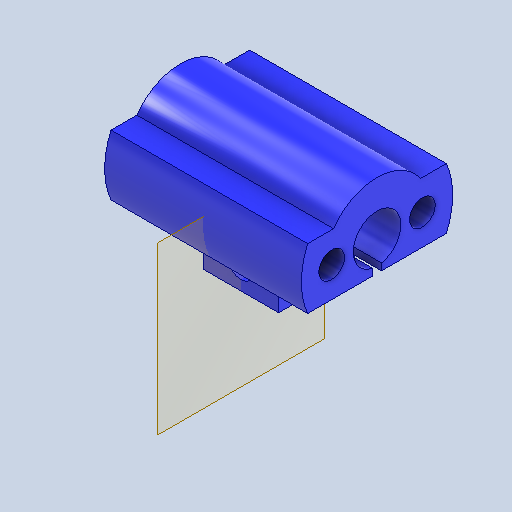
# Autodesk Inventor part: セットカラ―
Saved by Autodesk Inventor 2024 (Build 280153000, 153)
## iProperties
Created: 2020-01-17
Part Number: セットカラ―
Material: ABS プラスチック
Document SubType Name: Modeling
Designer: Hagihara Yuya
Density: 1.06 g/cm^3
Appearance: 青 - 壁塗料 - 光沢
Author: Hagihara Yuya
Autodesk Inventor part; units mm, degrees
ref_plane "YZ Plane" through (0, 0, 0) normal (1, 0, 0) x (0, 1, 0)
ref_plane "XZ Plane" through (0, 0, 0) normal (0, 1, 0) x (-1, 0, 0)
ref_plane "XY Plane" through (0, 0, 0) normal (0, 0, 1) x (1, 0, 0)
sketch "スケッチ1" plane through (0, 0, 0) normal (1, 0, 0) x (0, 1, 0)
  circle A0 centre (0, 0) radius 3.15
  circle A1 centre (0, 0) radius 7
  line L0 (0, 5) -> (-10, 5)
  line L1 (-10, 5) -> (-10, -5)
  line L2 (-10, -5) -> (0, -5)
  line L3 (0, -5) -> (0, 5) construction
  line L4 (-10, 0.6) -> (0, 0.6)
  line L5 (0, 0.6) -> (0, -0.6)
  line L6 (0, -0.6) -> (-10, -0.6)
  line L7 (-10, -0.6) -> (-10, 0.6)
  line L8 (4, 10) -> (-4, 10) construction
  line L9 (-4, 10) -> (-4, -10)
  line L10 (-4, -10) -> (4, -10) construction
  line L11 (4, -10) -> (4, 10)
  line L12 (4, 10) -> (-4, -10) construction
  line L13 (-4, 10) -> (4, -10) construction
  arc A2 (4, 9.1652) -> (-4, 9.1652) centre (0, 0) ccw
  arc A3 (-4, -9.1652) -> (4, -9.1652) centre (0, 0) ccw
  point P0 (-11, 3.3541)
  point P1 (-11, -3.3541)
  point P2 (-4.899, 5)
  point P3 (-4.899, -5)
  point P4 (-3.0923, 0.6)
  point P5 (-3.0923, -0.6)
  point P6 (-6.9742, -0.6)
  point P7 (-6.9742, 0.6)
  point P8 (0, -3.15)
  point P9 (0, 3.15)
  point P10 (0, 0.6)
  point P11 (-4, -5)
  point P12 (4, -5.7446)
  point P13 (4, 5.7446)
  point P14 (-4, 5)
  dimension "d0" = 6.3
  dimension "d1" = 14
  dimension "d2" = 5
  dimension "d3" = 5
  dimension "d4" = 10
  dimension "d18" = 1.2
  dimension "d19" = 0.6
  dimension "d45" = 8
  dimension "d46" = 20
  constraints: 28 end point, 6 parallel, 6 point on line, 4 centre point, 4 coincident, 4 point on circle, 3 horizontal, 3 midpoint, 3 perpendicular, 2 tangent
  measures "d0" diameter of A0
  measures "d1" diameter of A1
  measures "d2" distance from line of L2 point (0, 0)
  measures "d3" distance from line of point (0, 0) L0
  measures "d4" distance of L1.end L2.end
  measures "d18" distance between parallel lines of L4 L6
  measures "d19" distance from line of point (0, 0) L6
  measures "d45" distance of L9.end L10.end
  measures "d46" distance of L8.end L9.end
extrude "押し出し1" add sketch "スケッチ1" along normal blind 10 contours A0 L4 L9 A1 L11 L6 | L4 A1 L0 L9 | L9 L2 A1 L6 | L4 L1 L0 A1 | A1 L2 L1 L6 | L9 A2 L11 A1 | A1 L11 A3 L9 | A1 L11
sketch "スケッチ2" plane through (10, 0, 0) normal (1, 0, 0) x (0, 0, -1)
  line L0 (14, 0) -> (-14, 0) projected
  point P0 (0, 0)
  point P1 (-6, 0)
  point P2 (6, 0)
  dimension "d7" = 6
  dimension "d8" = 6
  constraints: 2 point on line
  measures "d7" distance of point (6, 0) point (0, 0)
  measures "d8" distance of point (-6, 0) point (0, 0)
hole "穴1" at (10, 0, 6) at (10, 0, -6) direction (-1, 0, 0) diameter 3.4 end through all counterbore diameter 6.5 counterbore depth 4
sketch "スケッチ3" plane through (0, -4.899, 5) normal (0, 0, 1) x (1, 0, 0)
  line L0 (0, -5.101) -> (10, -5.101) projected
  point P0 (5, -2.101)
  point P1 (5, -5.101)
  dimension "d44" = 3
  constraints: 1 midpoint, 1 vertical alignment
  measures "d44" distance from line of L0 point (5, -2.101)
hole "穴2" at (5, -7, 5) direction (0, 0, -1) diameter 3.4 end through all
sketch "スケッチ7" plane through (0, 0, 0) normal (-1, 0, 0) x (0, 0, 1)
  arc A0 (5.7446, 4) -> (-5.7446, 4) centre (0, 0) ccw projected
  arc A1 (5.7446, 4) -> (-5.7446, 4) centre (0, 0) ccw
  arc A2 (9.1652, -4) -> (9.1652, 4) centre (0, 0) ccw projected
  circle A3 centre (0, 0) radius 10
  line L0 (9.1652, 4) -> (-9.1652, 4)
  line L1 (-9.1652, -4) -> (9.1652, -4)
  line L2 (5, -10) -> (0.6, -10) projected
  line L3 (5, -10) -> (5, -4)
  line L4 (-5, -10) -> (-5, -4) projected
  line L5 (5, -10) -> (-5, -10)
  line L6 (-5, -10) -> (-5, -4)
  line L7 (-5, -4) -> (-5, -10)
  arc A4 (0.6, -3.0923) -> (-0.6, -3.0923) centre (0, 0) ccw projected
  circle A5 centre (0, 0) radius 3.15
  circle A6 centre (6, 0) radius 1.7 projected
  circle A7 centre (6, 0) radius 1.7
  circle A8 centre (-6, 0) radius 1.7 projected
  circle A9 centre (-6, 0) radius 1.7
  line L8 (-0.6, -3.0923) -> (-0.6, -4)
  line L9 (0.6, -10) -> (0.6, -3.0923) projected
  line L10 (0.6, -4) -> (0.6, -3.0923)
  point P0 (0.6, -3.0923)
  point P1 (-0.6, -3.0923)
  point P2 (-5.7446, 4)
  constraints: 16 end point, 6 point on line, 5 centre point, 5 coincident, 5 point on circle, 4 perpendicular, 2 collinear, 1 horizontal, 1 parallel
extrude "押し出し5" add sketch "スケッチ7" along normal blind 8 contours L0 A0 | L0 A2 L1 L9 A4 L8 A3
ref_plane "作業平面1" through (5, -10, 5) normal (1, 0, 0) x (0, 1, 0)
mirror "ミラー1" about plane through (5, -10, 5) normal (1, 0, 0) of "押し出し5"
equation "\"d3\" = d2"
equation "\"d19\" = 0.5 * d18"
equation "\"d8\" = d7"
